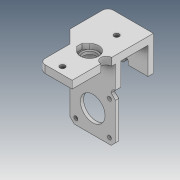
# Autodesk Inventor part: body
Saved by Autodesk Inventor 2021 (Build 250183000, 183)
## iProperties
Created: 2023-03-20
Part Number: body
Material: Generic
Document SubType Name: Modeling
Designer: WubbGmbaa
Density: 1 g/cm^3
Appearance: Default
Author: WubbGmbaa
Autodesk Inventor part; units mm, degrees
ref_plane "YZ Plane" through (0, 0, 0) normal (1, 0, 0) x (0, 1, 0)
ref_plane "XZ Plane" through (0, 0, 0) normal (0, 1, 0) x (-1, 0, 0)
ref_plane "XY Plane" through (0, 0, 0) normal (0, 0, 1) x (1, 0, 0)
sketch "Sketch1" plane through (0, 0, 0) normal (0, 1, 0) x (-1, 0, 0)
  line L0 (30, 0) -> (30, -75) construction
  line L1 (30, -75) -> (0, -75) construction
  line L2 (0, -75) -> (0, 0) construction
  line L3 (0, 0) -> (15.4, 0) construction
  line L4 (15.4, 0) -> (15.4, -6.5) construction
  line L5 (15.4, -6.5) -> (0, -6.5) construction
  line L6 (0, -6.5) -> (0, 0) construction
  line L7 (15.4, -6.5) -> (15.4, -31.5) construction
  circle A0 centre (15.4, -31.5) radius 8.5 construction
  line L8 (15.4, -31.5) -> (15.4, -56.5) construction
  circle A1 centre (15.4, -6.5) radius 2.35
  circle A2 centre (15.4, -56.5) radius 2.35
  line L9 (15.4, -23) -> (24.9, -23) construction
  line L10 (24.9, -23) -> (24.9, -40) construction
  line L11 (24.9, -40) -> (15.4, -40) construction
  line L12 (15.4, -40) -> (15.4, -23) construction
  line L13 (5.9, -29) -> (24.9, -29) construction
  line L14 (24.9, -29) -> (24.9, -34) construction
  line L15 (24.9, -34) -> (5.9, -34) construction
  line L16 (5.9, -34) -> (5.9, -29) construction
  line L17 (5.9, -29) -> (24.9, -34) construction
  line L18 (24.9, -29) -> (5.9, -34) construction
  line L19 (24.9, -29) -> (24.9, -34)
  line L20 (24.9, -29) -> (21.4283, -25.5075)
  line L21 (24.9, -34) -> (21.4283, -37.4925)
  arc A3 (21.4283, -25.5075) -> (21.4283, -37.4925) centre (15.4, -31.5) ccw
  arc A4 (0, -36.5) -> (0, -26.5) centre (0, -31.5) ccw
  line L22 (0, 0) -> (0, -26.5)
  line L23 (0, -36.5) -> (0, -75)
  line L24 (42, -40) -> (0, -40) construction
  line L25 (0, -40) -> (0, -75) construction
  line L26 (42, -40) -> (30, -40) construction
  line L27 (30, -40) -> (30, -28) construction
  line L28 (30, -28) -> (42, -28) construction
  line L29 (42, -28) -> (42, -40) construction
  line L30 (30, -28) -> (42, -40)
  line L31 (0, 0) -> (30, 0)
  line L32 (30, -28) -> (30, 0)
  line L33 (42, -40) -> (42, -75)
  line L34 (42, -75) -> (0, -75)
  dimension "d0" = 30
  dimension "d1" = 75
  dimension "d2" = 15.4
  dimension "d3" = 6.5
  dimension "d4" = 25
  dimension "d5" = 17
  dimension "d6" = 25
  dimension "d7" = 4.7
  dimension "d8" = 4.7
  dimension "d9" = 9.5
  dimension "d10" = 5
  dimension "d11" = 5
  dimension "d12" = 42
  dimension "d13" = 35
  dimension "d14" = 12
  constraints: 70 end point, 9 parallel, 9 point on circle, 6 point on line, 5 centre point, 5 collinear, 5 perpendicular, 4 coincident, 4 horizontal, 3 vertical, 2 midpoint, 2 tangent, 1 concentric
  measures "d0" distance of L0.end L1.end
  measures "d1" distance of L0.start L0.end
  measures "d2" distance of L4.end L5.end
  measures "d3" distance of L3.end L4.end
  measures "d4" distance of L4.end L7.end
  measures "d5" diameter of A0
  measures "d6" distance of L8.start L8.end
  measures "d7" diameter of A1
  measures "d8" diameter of A2
  measures "d9" distance of L10.end L11.end
  measures "d10" distance of L13.end L14.end
  measures "d11" radius of A4
  measures "d12" distance of L24.end L24.start
  measures "d13" distance of L24.start L33.end
  measures "d14" distance of L26.end L27.end
extrude "Extrusion1" add sketch "Sketch1" against normal blind 7
sketch "Sketch2" plane through (0, -7, 0) normal (0, -1, 0) x (1, 0, 0)
  circle A0 centre (-15.4, -6.5) radius 2.35 construction
  circle A1 centre (-15.4, -56.5) radius 2.35 construction
  line L0 (-15.4, -6.5) -> (-15.4, -10.75) construction
  line L1 (-15.4, -56.5) -> (-15.4, -52.25) construction
  line L2 (-15.4, -10.75) -> (-19.0806, -8.625)
  line L3 (-19.0806, -8.625) -> (-19.0806, -4.375)
  line L4 (-19.0806, -4.375) -> (-15.4, -2.25)
  line L5 (-15.4, -2.25) -> (-11.7194, -4.375)
  line L6 (-11.7194, -4.375) -> (-11.7194, -8.625)
  line L7 (-11.7194, -8.625) -> (-15.4, -10.75)
  line L8 (-15.4, -52.25) -> (-11.7194, -54.375)
  line L9 (-11.7194, -54.375) -> (-11.7194, -58.625)
  line L10 (-11.7194, -58.625) -> (-15.4, -60.75)
  line L11 (-15.4, -60.75) -> (-19.0806, -58.625)
  line L12 (-19.0806, -58.625) -> (-19.0806, -54.375)
  line L13 (-19.0806, -54.375) -> (-15.4, -52.25)
  point P0 (0, 0)
  dimension "d18" = 4.25
  dimension "d19" = 4.25
  constraints: 28 end point, 2 coincident, 2 vertical, 26 other
  measures "d18" distance of L0.start L0.end
  measures "d19" distance of L1.start L1.end
extrude "Extrusion2" cut sketch "Sketch2" against normal blind 3.5
sketch "Sketch3" plane through (0, -7, 0) normal (0, -1, 0) x (1, 0, 0)
  arc A0 (-21.4283, -37.4925) -> (-21.4283, -25.5075) centre (-15.4, -31.5) ccw projected
  circle A1 centre (-15.4, -31.5) radius 6
  line L0 (-24.9, -29) -> (-21.4283, -25.5075) projected
  line L1 (-24.9, -34) -> (-24.9, -29) projected
  line L2 (-21.4283, -37.4925) -> (-24.9, -34) projected
  point P0 (0, 0)
  dimension "d22" = 12
  constraints: 1 centre point, 1 coincident
  measures "d22" diameter of A1
extrude "Extrusion3" add sketch "Sketch3" against normal blind 2.1
sketch "Sketch4" plane through (0, -4.9, 0) normal (0, 1, 0) x (1, 0, 0)
  circle A0 centre (-15.4, 31.5) radius 6 projected
  circle A1 centre (-15.4, 31.5) radius 8
  point P0 (0, 0)
  dimension "d25" = 16
  constraints: 1 centre point, 1 coincident
  measures "d25" diameter of A1
extrude "Extrusion4" add sketch "Sketch4" along normal blind 0.5
sketch "Sketch5" plane through (0, -7, 0) normal (0, -1, 0) x (1, 0, 0)
  line L0 (0, -75) -> (0, -36.5) construction
  line L1 (-42, -70) -> (-42, -40) construction
  line L2 (0, -75) -> (-42, -75) construction
  line L3 (-42, -75) -> (-42, -40) construction
  line L4 (-42, -40) -> (0, -40) construction
  line L5 (0, -40) -> (0, -75) construction
  line L6 (0, -40) -> (-42, -40) construction
  line L7 (-42, -40) -> (-42, -45) construction
  line L8 (-42, -45) -> (0, -45) construction
  line L9 (0, -45) -> (0, -40) construction
  line L10 (-42, -40) -> (-37, -40) construction
  line L11 (-37, -40) -> (-37, -75) construction
  line L12 (-37, -75) -> (-42, -75) construction
  line L13 (-42, -75) -> (-42, -40) construction
  line L14 (-42, -75) -> (0, -75) construction
  line L15 (0, -75) -> (0, -70) construction
  line L16 (0, -70) -> (-42, -70) construction
  line L17 (-42, -70) -> (-42, -75) construction
  line L18 (-37, -75) -> (0, -75) projected
  line L19 (0, -75) -> (0, -70)
  line L20 (-37, -70) -> (0, -70)
  line L21 (-37, -45) -> (-37, -70)
  line L22 (0, -40) -> (-42, -40)
  line L23 (0, -45) -> (0, -40)
  line L24 (-37, -45) -> (0, -45)
  line L25 (-42, -40) -> (-42, -75) projected
  line L26 (-42, -40) -> (-42, -75)
  line L27 (-42, -75) -> (0, -75)
  point P0 (0, 0)
  dimension "d28" = 5
  dimension "d29" = 5
  constraints: 48 end point, 8 parallel, 6 perpendicular, 4 horizontal, 4 point on line, 3 collinear, 1 vertical
  measures "d28" distance of L7.end L6.end
  measures "d29" distance of L15.end L14.end
extrude "Extrusion5" add sketch "Sketch5" along normal blind 25
sketch "Sketch6" plane through (-42, -7, -40) normal (0, 0, 1) x (1, 0, 0)
  line L0 (5, -25) -> (42, -25) projected
  line L1 (38, -25) -> (0, -25)
  line L2 (0, -25) -> (0, -63)
  line L3 (4, -67) -> (38, -67)
  line L4 (42, -63) -> (42, -29)
  line L5 (42, -63) -> (38, -67)
  line L6 (4, -67) -> (0, -63)
  line L7 (42, -29) -> (38, -25)
  circle A0 centre (21, -46) radius 11.4
  line L8 (36.5, -61.5) -> (5.5, -61.5) construction
  line L9 (5.5, -61.5) -> (5.5, -30.5) construction
  line L10 (5.5, -30.5) -> (36.5, -30.5) construction
  line L11 (36.5, -30.5) -> (36.5, -61.5) construction
  line L12 (36.5, -61.5) -> (5.5, -30.5) construction
  line L13 (5.5, -61.5) -> (36.5, -30.5) construction
  circle A1 centre (36.5, -61.5) radius 1.8
  circle A2 centre (5.5, -61.5) radius 1.8
  circle A3 centre (5.5, -30.5) radius 1.8
  circle A4 centre (36.5, -30.5) radius 1.8
  point P0 (42, 7)
  point P1 (0, -67)
  point P2 (42, -67)
  dimension "d32" = 42
  dimension "d33" = 42
  dimension "d34" = 4
  dimension "d35" = 4
  dimension "d36" = 4
  dimension "d37" = 4
  dimension "d38" = 4
  dimension "d39" = 4
  dimension "d40" = 22.8
  dimension "d41" = 31
  dimension "d42" = 31
  dimension "d43" = 3.6
  dimension "d44" = 3.6
  dimension "d45" = 3.6
  dimension "d46" = 3.6
  constraints: 26 end point, 6 point on line, 5 centre point, 4 coincident, 4 parallel, 2 horizontal, 2 midpoint, 2 perpendicular
  measures "d32" distance of point (42, -67) point (0, -67)
  measures "d33" distance of point (0, -67) L1.end
  measures "d34" distance of L4.start point (42, -67)
  measures "d35" distance of L3.end point (42, -67)
  measures "d36" distance of L3.start point (0, -67)
  measures "d37" distance of L2.end point (0, -67)
  measures "d38" distance of L4.end L0.end
  measures "d39" distance of L1.start L0.end
  measures "d40" diameter of A0
  measures "d41" distance of L9.end L10.end
  measures "d42" distance of L8.end L9.end
  measures "d43" diameter of A1
  measures "d44" diameter of A2
  measures "d45" diameter of A3
  measures "d46" diameter of A4
extrude "Extrusion6" add sketch "Sketch6" against normal blind 3
sketch "Sketch7" plane through (-42, -7, -40) normal (0, 0, 1) x (1, 0, 0)
  line L0 (42, -25) -> (38, -25) projected
  arc A0 (42, -21) -> (38, -25) centre (42, -25) ccw
  line L1 (42, -21) -> (42, -25)
  point P0 (42, 7)
  constraints: 2 end point, 2 point on circle, 1 centre point, 1 vertical
extrude "Extrusion7" cut sketch "Sketch7" against normal blind 5
sketch "Sketch8" plane through (0, 0, -75) normal (0, 0, -1) x (-1, 0, 0)
  line L0 (42, -32) -> (0, -32) construction
  line L1 (20.5, -34.5) -> (20.5, -29.5) construction
  line L2 (37, -32) -> (4, -32) construction
  line L3 (23, -34.5) -> (23, -29.5) construction
  line L4 (18, -29.5) -> (18, -34.5) construction
  arc A0 (18, -34.5) -> (23, -34.5) centre (20.5, -34.5) ccw construction
  arc A1 (23, -29.5) -> (18, -29.5) centre (20.5, -29.5) ccw construction
  line L5 (20.5, -32) -> (25.5, -32) construction
  arc A2 (23, -29.5) -> (18, -29.5) centre (20.5, -29.5) ccw
  line L6 (23, -29.5) -> (23, -32)
  line L7 (18, -29.5) -> (18, -32)
  line L8 (18, -32) -> (23, -32)
  point P0 (0, 0)
  dimension "d51" = 2.5
  dimension "d52" = 90
  dimension "d53" = 5
  constraints: 16 end point, 7 point on circle, 4 midpoint, 4 tangent, 3 centre point, 2 perpendicular, 1 coincident, 1 collinear, 1 horizontal, 1 parallel
  measures "d51" distance of L5.start L1.end
  measures "d52" angle of L5 L1
  measures "d53" diameter of A1
extrude "Extrusion8" cut sketch "Sketch8" against normal blind 5
sketch "Sketch9" plane through (-42, -7, -43) normal (0, 0, -1) x (-1, 0, 0)
  line L0 (0, -25) -> (-19, -25) construction
  line L1 (0, -25) -> (-4, -25) construction
  line L2 (-4, -25) -> (-4, -29) construction
  line L3 (-4, -29) -> (0, -29) construction
  line L4 (0, -29) -> (0, -25) construction
  line L5 (0, -29) -> (-4, -25)
  line L6 (0, -25) -> (-4, -25)
  line L7 (0, -25) -> (0, -29)
  line L8 (0, 0) -> (0, -63) projected
  point P0 (-42, 7)
  dimension "d56" = 4
  dimension "d57" = 4
  constraints: 14 end point, 2 collinear, 2 parallel, 1 horizontal, 1 perpendicular
  measures "d56" distance of L3.end L2.end
  measures "d57" distance of L2.end L1.end
extrude "Extrusion9" add sketch "Sketch9" along normal up to surface (32 mm away)
fillet "Fillet1" radius 5 2 edges at (-30, -3.5, 0) (-42, -18, -75)
equation "\"d35\" = d34"
equation "\"d36\" = d34"
equation "\"d37\" = d36"
equation "\"d38\" = d34"
equation "\"d39\" = d38"
body "Solid1"
